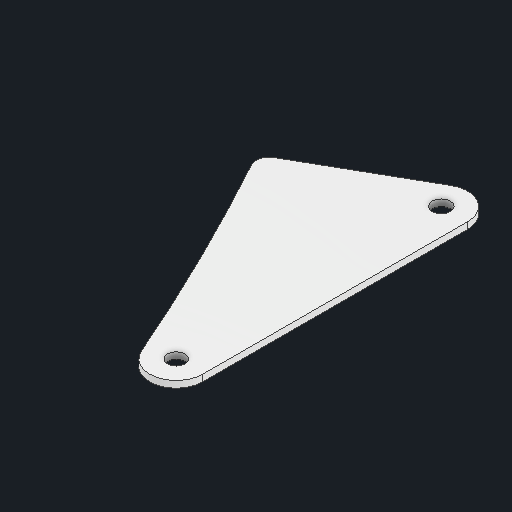
# Autodesk Inventor part: Magazine Gusset
Saved by Autodesk Inventor 2025 (Build 290162000, 162)
## iProperties
Created: 2024-12-31
Part Number: Magazine Gusset
Material: Acetal Resin, White
Document SubType Name: Modeling
Designer: Averey Ku
Density: 1.425 g/cm^3
Appearance: Smooth - White
Author: Averey Ku
Autodesk Inventor part; units mm, degrees
ref_plane "YZ Plane" through (0, 0, 0) normal (1, 0, 0) x (0, 1, 0)
ref_plane "XZ Plane" through (0, 0, 0) normal (0, 1, 0) x (-1, 0, 0)
ref_plane "XY Plane" through (0, 0, 0) normal (0, 0, 1) x (1, 0, 0)
sketch "main" plane through (0, 0, 0) normal (0, 0, 1) x (1, 0, 0)
  circle A0 centre (31.4944, -42.9627) radius 2.1844
  arc A1 (31.4944, -49.3127) -> (37.0053, -39.8078) centre (31.4944, -42.9627) ccw
  arc A2 (-34.551, -37.1452) -> (-32.0056, -49.3127) centre (-32.0056, -42.9627) ccw
  arc A3 (-34.551, -37.1452) -> (17.2626, -11.6066) centre (-289.0911, 544.606) ccw
  line L0 (37.0053, -39.8078) -> (21.5498, -12.8103)
  line L1 (-32.0056, -49.3127) -> (31.4944, -49.3127)
  arc A4 (21.5498, -12.8103) -> (17.2626, -11.6066) centre (18.7944, -14.3877) ccw
  circle A5 centre (-32.0056, -42.9627) radius 2.0955
  point P0 (5.1717, -33.3366)
  point P1 (19.9944, -10.0932)
  dimension "d0" = 1270
  dimension "d1" = 12.7
  dimension "d2" = 12.7
  dimension "d3" = 3.175
  dimension "d4" = 4.191
  dimension "d7" = 34.925
  dimension "d8" = 12.7
  measures "d0" diameter of A3
  measures "d1" diameter of A2
  measures "d2" diameter of A1
  measures "d3" radius of A4
  measures "d4" diameter of A5
  measures "d7" distance from line of L1 A4.centre
  measures "d8" horizontal distance of A0.centre A4.centre
sketch "Sketch1" plane through (0, 0, 0) normal (0, 1, 0) x (-1, 0, 0)
  circle A0 centre (-0.1035, -63.4999) radius 2.1844
  arc A1 (-6.4535, -63.4896) -> (3.0424, -69.0159) centre (-0.1035, -63.4999) ccw
  arc A2 (5.8217, 2.5359) -> (-6.35, 0.0103) centre (0, 0) ccw
  arc A3 (5.8217, 2.5359) -> (31.2757, -49.3193) centre (587.9868, 256.1277) ccw
  line L0 (3.0424, -69.0159) -> (30.0651, -53.6045)
  line L1 (-6.35, 0.0103) -> (-6.4535, -63.4896)
  arc A4 (30.0651, -53.6045) -> (31.2757, -49.3193) centre (28.4922, -50.8465) ccw
  circle A5 centre (0, 0) radius 2.0955
  point P0 (0, 0)
  constraints: 1 other
extrude "Extrusion1" add sketch "Sketch1" along normal blind 1.5875
body "Solid1"
